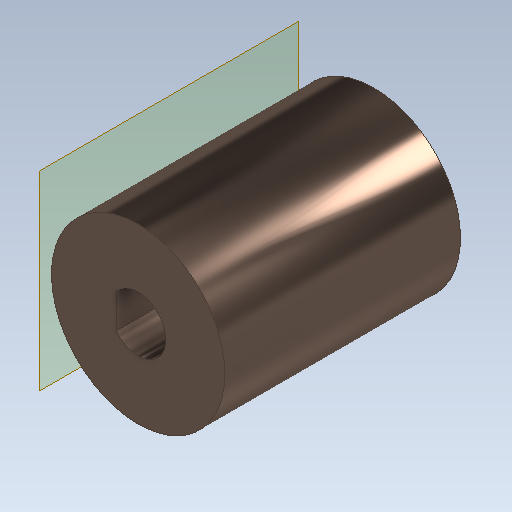
# Autodesk Inventor part: nmrv-50 to megatroque motor coupler
Saved by Autodesk Inventor 2020 (Build 240168000, 168)
## iProperties
Created: 2020-08-02
Part Number: nmrv-50 to megatroque motor coupler
Material: Generic
Document SubType Name: Modeling
Designer: Vikki
Density: 1 g/cm^3
Appearance: Gunmetal - Antique Polished
Author: Vikki
Autodesk Inventor part; units mm, degrees
ref_plane "YZ Plane" through (0, 0, 0) normal (1, 0, 0) x (0, 1, 0)
ref_plane "XZ Plane" through (0, 0, 0) normal (0, 1, 0) x (-1, 0, 0)
sketch "Sketch1" plane through (0, 0, 0) normal (0, 0, 1) x (1, 0, 0)
  circle A0 centre (0, 0) radius 6 projected
  line L0 (-7.6, 2) -> (-5.6569, 2) projected
  line L1 (-7.6, 2) -> (-7.6, -2) projected
  line L2 (-5.6569, -2) -> (-7.6, -2) projected
  circle A1 centre (0, 0) radius 12.5
  point P0 (0, 0)
  dimension "d0" = 25
  constraints: 1 centre point, 1 coincident
  measures "d0" diameter of A1
extrude "Extrusion1" add sketch "Sketch1" against normal blind 14
sketch "Sketch2" plane through (0, 0, 0) normal (0, 0, 1) x (1, 0, 0)
  arc A0 (19.4059, 4.8385) -> (16.8372, 10.794) centre (0, 0) ccw projected
  circle A1 centre (0, 0) radius 12.5 projected
  point P0 (0, 0)
extrude "Extrusion2" add sketch "Sketch2" along normal blind 8
sketch "Sketch3" plane through (0, 0, 8) normal (0, 0, 1) x (1, 0, 0)
  circle A0 centre (0, 0) radius 12.5 projected
  line L0 (-3.175, -2.433) -> (-3.175, 2.433) projected
  arc A1 (-3.175, -2.433) -> (-3.175, 2.433) centre (0, 0) ccw projected
  point P0 (0, 0)
extrude "Extrusion3" add sketch "Sketch3" along normal blind 12
ref_plane "Work Plane2" through (-12.5, 0, 0) normal (-1, 0, 0) x (0, -1, 0)
ref_plane "Work Plane1" through (-3.175, -2.433, 10) normal (-1, 0, 0) x (0, 1, 0)
sketch "Sketch4" plane through (-12.5, 0, 0) normal (-1, 0, 0) x (0, -1, 0)
  circle A0 centre (0, 12) radius 3
  line L0 (12.5, 20) -> (-12.5, 20) projected
  point P0 (0, 0)
  dimension "d7" = 8
  dimension "d8" = 6
  constraints: 1 centre point, 1 vertical alignment
  measures "d7" distance from line of L0 A0.centre
  measures "d8" diameter of A0
ref_plane "Work Plane3" through (-3.175, -2.433, 10) normal (-1, 0, 0) x (0, 0, 1)
extrude "Extrusion4" cut sketch "Sketch4" against normal up to surface (9.325 mm away)
thread "Thread1" size "M6x1" class "6H" standard "ANSI Metric M Profile" length 20
body "Solid1"
